Autodesk Fusion 360 part; units mm, degrees
note: some values were not read from the file. Chosen so that the rebuilt part matches the saved one: which bodies a step acts on. Set by a fixed rule: which sketch regions a step uses.
(part 3 of 3)
sketch "Esquisse40" plane through (480, 0, 0) normal (1, 0, 0) x (0, 0, -1)
  line L0 (-510, -15) -> (-510, -115)
  line L1 (-510, -115) -> (-540, -115)
  line L2 (-540, -115) -> (-540, -165)
  line L3 (-540, -165) -> (-950, -165)
  line L4 (-950, -165) -> (-950, -115)
  line L5 (-950, -115) -> (-980, -115)
  line L6 (-980, -115) -> (-980, -15)
  line L7 (-980, -15) -> (-510, -15)
  line L8 (-500, -185) -> (-500, 20)
  line L9 (-500, 20) -> (-1000, 20)
  line L10 (-1000, 20) -> (-1000, -185)
  line L11 (-1000, -185) -> (-500, -185)
  circle A0 centre (-965.0414, -132.162) radius 10.681
  circle A1 centre (-525, -132.162) radius 10.323
extrude "Extrusion42" cut sketch "Esquisse40" against normal blind 10 contours A0 | A1 bodies 33
sketch "Esquisse41" plane through (0, -15, 0) normal (0, -1, 0) x (1, 0, 0)
  line L0 (480, 980) -> (20, 980)
  line L1 (20, 980) -> (20, 510)
  line L2 (20, 510) -> (480, 510)
  line L3 (480, 510) -> (480, 980)
  line L4 (450, 510) -> (480, 510)
  line L5 (480, 510) -> (480, 540)
  line L6 (480, 540) -> (450, 540)
  line L7 (450, 540) -> (450, 510)
  line L8 (450, 950) -> (480, 950)
  line L9 (480, 950) -> (480, 980)
  line L10 (480, 980) -> (450, 980)
  line L11 (450, 980) -> (450, 950)
  constraint horizontal L4
  constraint vertical L5
  constraint horizontal L6
  constraint vertical L7
  constraint coincident L3 L5.end
  constraint coincident L2 L4.start
  constraint horizontal L8
  constraint vertical L9
  constraint horizontal L10
  constraint vertical L11
  constraint coincident L0.start L3.end
extrude "Extrusion43" add sketch "Esquisse41" along normal blind 50 contours L0 L3 L8 L9 L10 L11 | L2 L3 L4 L5 L6 L7 bodies 33
sketch "Esquisse42" plane through (480, 0, 0) normal (1, 0, 0) x (0, 0, -1)
  circle A0 centre (-525, -132.162) radius 10.323
  circle A1 centre (-965.0414, -132.162) radius 10.681
  line L0 (-510, -65) -> (-510, -115)
  line L1 (-510, -115) -> (-540, -115)
  line L2 (-540, -115) -> (-540, -165)
  line L3 (-540, -165) -> (-950, -165)
  line L4 (-950, -165) -> (-950, -115)
  line L5 (-950, -115) -> (-980, -115)
  line L6 (-980, -115) -> (-980, -65)
  line L7 (-980, -65) -> (-950, -65)
  line L8 (-950, -65) -> (-950, -15)
  line L9 (-950, -15) -> (-540, -15)
  line L10 (-540, -15) -> (-540, -65)
  line L11 (-540, -65) -> (-510, -65)
  line L12 (-500, -185) -> (-500, 20)
  line L13 (-500, 20) -> (-1000, 20)
  line L14 (-1000, 20) -> (-1000, -185)
  line L15 (-1000, -185) -> (-500, -185)
  circle A2 centre (-521.5285, -34.781) radius 9.6789
  circle A3 centre (-964.5674, -34.781) radius 10.3156
extrude "Extrusion44" cut sketch "Esquisse42" against normal blind 10 contours A2 | A3 bodies 33
sketch "Esquisse43" plane through (0, -165, 0) normal (0, 1, 0) x (-1, 0, 0)
  line L0 (-450, 980) -> (-450, 950)
  line L1 (-450, 950) -> (-480, 950)
  line L2 (-480, 950) -> (-480, 540)
  line L3 (-480, 540) -> (-450, 540)
  line L4 (-450, 540) -> (-450, 510)
  line L5 (-450, 510) -> (-20, 510)
  line L6 (-20, 510) -> (-20, 980)
  line L7 (-20, 980) -> (-450, 980)
  line L8 (-450, 760) -> (-480, 760)
  line L9 (-480, 760) -> (-480, 730)
  line L10 (-480, 730) -> (-450, 730)
  line L11 (-450, 730) -> (-450, 760)
  constraint horizontal L8
  constraint vertical L9
  constraint horizontal L10
  constraint vertical L11
  constraint coincident L2 L9.end
extrude "Extrusion45" add sketch "Esquisse43" along normal blind 50 contours L2 L8 L9 L10 L11 bodies 33
sketch "Esquisse44" plane through (480, 0, 0) normal (1, 0, 0) x (0, 0, -1)
  circle A0 centre (-964.5674, -34.781) radius 10.3156
  circle A1 centre (-521.5285, -34.781) radius 9.6789
  circle A2 centre (-525, -132.162) radius 10.323
  circle A3 centre (-965.0414, -132.162) radius 10.681
  line L0 (-510, -65) -> (-510, -115)
  line L1 (-510, -115) -> (-540, -115)
  line L2 (-540, -115) -> (-540, -165)
  line L3 (-540, -165) -> (-730, -165)
  line L4 (-730, -165) -> (-730, -115)
  line L5 (-730, -115) -> (-760, -115)
  line L6 (-760, -115) -> (-760, -165)
  line L7 (-760, -165) -> (-950, -165)
  line L8 (-950, -165) -> (-950, -115)
  line L9 (-950, -115) -> (-980, -115)
  line L10 (-980, -115) -> (-980, -65)
  line L11 (-980, -65) -> (-950, -65)
  line L12 (-950, -65) -> (-950, -15)
  line L13 (-950, -15) -> (-540, -15)
  line L14 (-540, -15) -> (-540, -65)
  line L15 (-540, -65) -> (-510, -65)
  line L16 (-500, -185) -> (-500, 20)
  line L17 (-500, 20) -> (-1000, 20)
  line L18 (-1000, 20) -> (-1000, -185)
  line L19 (-1000, -185) -> (-500, -185)
  circle A4 centre (-745.3396, -137.266) radius 10.7846
extrude "Extrusion46" cut sketch "Esquisse44" against normal blind 10 contours A4 bodies 33
move_body "Déplacer6" bodies 14 to x (1, 0, 0) y (0, 1, 0) z (0, 0, 1) at (25, 0, 0)
sketch "Esquisse45" plane through (505, 0, 0) normal (-1, 0, 0) x (0, 0, 1)
  line L0 (500, 20) -> (500, -185)
  line L1 (500, -185) -> (1000, -185)
  line L2 (1000, -185) -> (1000, 20)
  line L3 (1000, 20) -> (500, 20)
  circle A0 centre (525, -125) radius 14.811
  circle A1 centre (975, -125) radius 11.6902
extrude "Extrusion47" cut sketch "Esquisse45" against normal blind 10 contours A0 | A1 bodies 14
sketch "Esquisse46" plane through (505, 0, 0) normal (-1, 0, 0) x (0, 0, 1)
  circle A0 centre (975, -125) radius 11.6902
  circle A1 centre (525, -125) radius 14.811
  line L0 (500, 20) -> (500, -185)
  line L1 (500, -185) -> (1000, -185)
  line L2 (1000, -185) -> (1000, 20)
  line L3 (1000, 20) -> (500, 20)
  circle A2 centre (515.6973, -40.3058) radius 11.1679
  circle A3 centre (988.0559, -36.5081) radius 10.5703
  circle A4 centre (700, -110) radius 11.5
  dimension "d185" = 23
  measures "d185" diameter of A4
extrude "Extrusion48" cut sketch "Esquisse46" against normal blind 10 contours A2 | A3 | A4 bodies 14
sketch "Esquisse47" plane through (505, 0, 0) normal (-1, 0, 0) x (0, 0, 1)
  circle A0 centre (700, -110) radius 11.5
  circle A1 centre (988.0559, -36.5081) radius 10.5703
  circle A2 centre (515.6973, -40.3058) radius 11.1679
  circle A3 centre (975, -125) radius 11.6902
  circle A4 centre (525, -125) radius 14.811
  line L0 (500, 20) -> (500, -185)
  line L1 (500, -185) -> (1000, -185)
  line L2 (1000, -185) -> (1000, 20)
  line L3 (1000, 20) -> (500, 20)
  line L4 (510, -95) -> (538.9521, -95)
  line L5 (538.9521, -95) -> (538.9521, -97.8044)
  line L6 (538.9521, -97.8044) -> (510, -97.8044)
  line L7 (510, -97.8044) -> (510, -95)
  line L8 (986, -107) -> (963, -107)
  line L9 (963, -107) -> (963, -108)
  line L10 (963, -108) -> (986, -108)
  line L11 (986, -108) -> (986, -107)
  constraint horizontal L4
  constraint vertical L5
  constraint horizontal L6
  constraint vertical L7
  constraint horizontal L8
  constraint vertical L9
  constraint horizontal L10
  constraint vertical L11
extrude "Extrusion49" add sketch "Esquisse47" along normal blind 20 contours L4 L5 L6 L7 | L8 L9 L10 L11 bodies 14
sketch "Esquisse48" plane through (505, 0, 0) normal (-1, 0, 0) x (0, 0, 1)
  line L0 (510, -97.8044) -> (510, -95)
  line L1 (510, -95) -> (538.9521, -95)
  line L2 (538.9521, -95) -> (538.9521, -97.8044)
  line L3 (538.9521, -97.8044) -> (510, -97.8044)
  line L4 (986, -108) -> (963, -108)
  line L5 (963, -108) -> (963, -107)
  line L6 (963, -107) -> (986, -107)
  line L7 (986, -107) -> (986, -108)
  circle A0 centre (700, -110) radius 11.5
  circle A1 centre (988.0559, -36.5081) radius 10.5703
  circle A2 centre (515.6973, -40.3058) radius 11.1679
  circle A3 centre (975, -125) radius 11.6902
  circle A4 centre (525, -125) radius 14.811
  line L8 (500, 20) -> (500, -185)
  line L9 (500, -185) -> (1000, -185)
  line L10 (1000, -185) -> (1000, 20)
  line L11 (1000, 20) -> (500, 20)
  line L12 (683, -94) -> (746, -94)
  line L13 (746, -94) -> (746, -91)
  line L14 (746, -91) -> (683, -91)
  line L15 (683, -91) -> (683, -94)
  constraint horizontal L12
  constraint vertical L13
  constraint horizontal L14
  constraint vertical L15
extrude "Extrusion50" add sketch "Esquisse48" along normal blind 20 contours L12 L13 L14 L15 bodies 14
move_body "Déplacer7" bodies 14 to x (1, 0, 0) y (0, 1, 0) z (0, 0, 1) at (170, 0, 0)
split "Scinder6" by plane through (480, -165, 1000) normal (1, 0, 0) bodies 32 makes body 34 at (500, 166.6667, 666.6667)
sketch "Esquisse49" plane through (0, 0, 500) normal (0, 0, -1) x (-1, 0, 0)
  line L0 (-480, 240) -> (-480, 20)
  line L1 (-480, 20) -> (-100, 20)
  line L2 (-100, 20) -> (-100, 240)
  line L3 (-100, 240) -> (-480, 240)
  line L4 (-475, 100) -> (-465, 100)
  line L5 (-460, 95) -> (-460, 25)
  line L6 (-465, 20) -> (-475, 20)
  line L7 (-480, 25) -> (-480, 95)
  arc A0 (-475, 100) -> (-480, 95) centre (-475, 95) ccw
  arc A1 (-460, 95) -> (-465, 100) centre (-465, 95) ccw
  arc A2 (-480, 25) -> (-475, 20) centre (-475, 25) ccw
  arc A3 (-465, 20) -> (-460, 25) centre (-465, 25) ccw
  dimension "d192" = 5
  constraint horizontal L4
  constraint vertical L5
  constraint horizontal L6
  constraint vertical L7
  constraint tangent L4 A0
  constraint tangent L7 A0
  constraint tangent L5 A1
  constraint tangent L4 A1
  constraint equal A0 A1
  constraint tangent L6 A2
  constraint tangent L7 A2
  constraint equal A0 A2
  constraint tangent L5 A3
  constraint tangent L6 A3
  constraint equal A0 A3
  measures "d192" radius of A0
extrude "Extrusion51" add sketch "Esquisse49" along normal blind 20 contours L0 L1 L4 L5 L6 L7 A0 A1 A2 A3 bodies 32 33 34
sketch "Esquisse50" plane through (0, 100, 0) normal (0, 1, 0) x (-1, 0, 0)
  line L0 (-465, 500) -> (-475, 500)
  line L1 (-475, 500) -> (-475, 480)
  line L2 (-475, 480) -> (-465, 480)
  line L3 (-465, 480) -> (-465, 500)
  circle A0 centre (-470, 490) radius 3
  dimension "d195" = 6
  measures "d195" diameter of A0
extrude "Extrusion52" add sketch "Esquisse50" along normal blind 20 contours A0 bodies 32
fillet "Congé1" radius 2.5 1 edges at (472.797, 120, 488.9152) on bodies 32
fillet "Congé2" radius 3 8 edges at (470, 20, 480) (461.4645, 21.4645, 480) (460, 60, 480) (461.4645, 98.5355, 480) (470, 100, 480) (478.5355, 98.5355, 480) (480, 60, 480) (478.5355, 21.4645, 480) on bodies 32
split "Scinder7" by plane through (0, 20, 0) normal (0, 1, 0) bodies 32 makes body 35 at (220.0253, 118.6227, 500)
split "Scinder8" by plane through (480, -165, 1000) normal (1, 0, 0) bodies 35 makes body 36 at (500, 166.6667, 666.6667)
sketch "Esquisse51" plane through (480, 0, 0) normal (1, 0, 0) x (0, 0, -1)
  line L0 (-483, 25) -> (-483, 95)
  line L1 (-483, 95) -> (-500, 95)
  line L2 (-500, 95) -> (-500, 240)
  line L3 (-500, 240) -> (-509, 240)
  line L4 (-509, 240) -> (-509, 20)
  line L5 (-509, 20) -> (-500, 20)
  line L6 (-500, 20) -> (-500, 25)
  line L7 (-500, 25) -> (-483, 25)
  line L8 (-500, 95) -> (-475.4609, 95)
  line L9 (-475.4609, 95) -> (-475.4609, -14.7189)
  line L10 (-475.4609, -14.7189) -> (-500, -14.7189)
  line L11 (-500, -14.7189) -> (-500, 95)
  line L12 (-500, 95) -> (-475.4609, 95)
  line L13 (-475.4609, 95) -> (-475.4609, 146.276)
  line L14 (-475.4609, 146.276) -> (-500, 146.276)
  line L15 (-500, 146.276) -> (-500, 95)
  constraint horizontal L8
  constraint vertical L9
  constraint horizontal L10
  constraint vertical L11
  constraint coincident L1.end L2.start
  constraint horizontal L12
  constraint vertical L13
  constraint horizontal L14
  constraint vertical L15
extrude "Extrusion53" cut sketch "Esquisse51" against normal blind 50 contours L0 L1 L7 L8 L11 L12 | L0 L6 L7 L8 L9 L10 L11 L12 | L1 L2 L8 L12 L13 L14 L15 bodies 35
hidden bodies 7 36
equation "d99 = ( 90 / 2 ) * 1 mm"
equation "d113 = ( 65 / 2 ) * 1 mm"
equation "d130 = 500 mm - 40 mm"
named bodies: "Faux plafond", "Sol", "Plaque avant faux plafond", "Pièce sans plafond", "Colonne à fils", "Murs (coffret)", "Sol (coffret)", "Plaque trouée (coffret)", "Ventilateur (coffret)", "Faux Plafond", "Plaque_avant_faux_plafond", "Plaque_droite_(ouvrante)", "Ventilo", "Grille", "Grille (1)", "Grille (2)", "Grille (3)", "Grille (4)", "Coffret_sans_plaque_droite", "Coffret_sans_plaque_ouvrante", "Piece_porte_droite_(ouvrante)", "Pièce_sans_plaque_droite", "Plaque_droite_Pièce_(ouvrante)"
